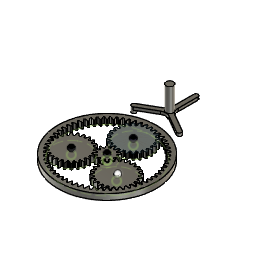
SizeFixedPlanetaryGearShaft (Autodesk Fusion 360 design; units mm, degrees)
description: Spur Gear; Diametrial Pitch: 10.0; Num Teeth: 60; Pressure Angle: 20.0; Backlash: 0.00 in
description: Spur Gear; Diametrial Pitch: 10.0; Num Teeth: 12; Pressure Angle: 20.0; Backlash: 0.00 in
description: Spur Gear; Diametrial Pitch: 10.0; Num Teeth: 24; Pressure Angle: 20.0; Backlash: 0.03 in
Autodesk Fusion 360 part; units mm, degrees
(part 1 of 3)
sketch "Sketch1" plane through (0, 0, 0) normal (0, 0, 1) x (1, 0, 0) in component "Spur Gear (60 teeth)"
  circle A0 centre (0, 0) radius 73.1012
  circle A1 centre (0, 0) radius 1.4986
extrude "Extrude1" add sketch "Sketch1" along normal blind 10.16 makes body 1 in component "Spur Gear (60 teeth)"
sketch "Sketch2" plane through (0, 0, 0) normal (0, 0, 1) x (1, 0, 0) in component "Spur Gear (60 teeth)"
  spline S0 degree 5 poles (71.5442, -2.941) (71.5649, -2.941) (71.6065, -2.9408) (71.6689, -2.94) (71.7521, -2.938) (71.8561, -2.9339) (71.96, -2.9282) (72.064, -2.921) (72.168, -2.9123) (72.272, -2.9022) (72.3759, -2.891) (72.4799, -2.8787) (72.5838, -2.8655) (72.6877, -2.8514) (72.7915, -2.8365) (72.8954, -2.8208) (72.9992, -2.8044) (73.1029, -2.7872) (73.2067, -2.7693) (73.3103, -2.7506) (73.414, -2.7311) (73.5176, -2.711) (73.6212, -2.6902) (73.7248, -2.6688) (73.8283, -2.6468) (73.9317, -2.6241) (74.0351, -2.6008) (74.1385, -2.577) (74.2418, -2.5525) (74.3451, -2.5275) (74.4484, -2.5019) (74.5516, -2.4757) (74.6547, -2.449) (74.7578, -2.4218) (74.8608, -2.394) (74.9638, -2.3657) (75.0668, -2.3369) (75.1697, -2.3075) (75.2725, -2.2777) (75.3753, -2.2474) (75.478, -2.2166) (75.5807, -2.1852) (75.6833, -2.1535) (75.7859, -2.1212) (75.8884, -2.0885) (75.9909, -2.0553) (76.0933, -2.0216) (76.1956, -1.9875) (76.2979, -1.953) (76.4001, -1.918) (76.5023, -1.8825) (76.6044, -1.8466) (76.7064, -1.8103) (76.8084, -1.7736) (76.9103, -1.7364) (77.0122, -1.6988) (77.114, -1.6608) (77.2157, -1.6223) (77.3174, -1.5835) (77.419, -1.5442) (77.5205, -1.5046) (77.622, -1.4645) (77.7234, -1.424) (77.8247, -1.3831) (77.926, -1.3419) (78.0272, -1.3002) (78.1283, -1.2582) (78.2294, -1.2157) (78.3304, -1.1729) (78.4313, -1.1297) (78.5322, -1.0862) (78.6128, -1.051) (78.6733, -1.0244) (78.7135, -1.0067) (78.7337, -0.9978) knots 0 0 0 0 0 0 0.01428571 0.02857143 0.04285714 0.05714286 0.07142857 0.08571429 0.1 0.11428571 0.12857143 0.14285714 0.15714286 0.17142857 0.18571429 0.2 0.21428571 0.22857143 0.24285714 0.25714286 0.27142857 0.28571429 0.3 0.31428571 0.32857143 0.34285714 0.35714286 0.37142857 0.38571429 0.4 0.41428571 0.42857143 0.44285714 0.45714286 0.47142857 0.48571429 0.5 0.51428571 0.52857143 0.54285714 0.55714286 0.57142857 0.58571429 0.6 0.61428571 0.62857143 0.64285714 0.65714286 0.67142857 0.68571429 0.7 0.71428571 0.72857143 0.74285714 0.75714286 0.77142857 0.78571429 0.8 0.81428571 0.82857143 0.84285714 0.85714286 0.87142857 0.88571429 0.9 0.91428571 0.92857143 0.94285714 0.95714286 0.97142857 0.98571429 1 1 1 1 1 1
  spline S1 degree 5 poles (71.5442, 2.941) (71.5649, 2.941) (71.6065, 2.9408) (71.6689, 2.94) (71.7521, 2.938) (71.8561, 2.9339) (71.96, 2.9282) (72.064, 2.921) (72.168, 2.9123) (72.272, 2.9022) (72.3759, 2.891) (72.4799, 2.8787) (72.5838, 2.8655) (72.6877, 2.8514) (72.7915, 2.8365) (72.8954, 2.8208) (72.9992, 2.8044) (73.1029, 2.7872) (73.2067, 2.7693) (73.3103, 2.7506) (73.414, 2.7311) (73.5176, 2.711) (73.6212, 2.6902) (73.7248, 2.6688) (73.8283, 2.6468) (73.9317, 2.6241) (74.0351, 2.6008) (74.1385, 2.577) (74.2418, 2.5525) (74.3451, 2.5275) (74.4484, 2.5019) (74.5516, 2.4757) (74.6547, 2.449) (74.7578, 2.4218) (74.8608, 2.394) (74.9638, 2.3657) (75.0668, 2.3369) (75.1697, 2.3075) (75.2725, 2.2777) (75.3753, 2.2474) (75.478, 2.2166) (75.5807, 2.1852) (75.6833, 2.1535) (75.7859, 2.1212) (75.8884, 2.0885) (75.9909, 2.0553) (76.0933, 2.0216) (76.1956, 1.9875) (76.2979, 1.953) (76.4001, 1.918) (76.5023, 1.8825) (76.6044, 1.8466) (76.7064, 1.8103) (76.8084, 1.7736) (76.9103, 1.7364) (77.0122, 1.6988) (77.114, 1.6608) (77.2157, 1.6223) (77.3174, 1.5835) (77.419, 1.5442) (77.5205, 1.5046) (77.622, 1.4645) (77.7234, 1.424) (77.8247, 1.3831) (77.926, 1.3419) (78.0272, 1.3002) (78.1283, 1.2582) (78.2294, 1.2157) (78.3304, 1.1729) (78.4313, 1.1297) (78.5322, 1.0862) (78.6128, 1.051) (78.6733, 1.0244) (78.7135, 1.0067) (78.7337, 0.9978) knots 0 0 0 0 0 0 0.01428571 0.02857143 0.04285714 0.05714286 0.07142857 0.08571429 0.1 0.11428571 0.12857143 0.14285714 0.15714286 0.17142857 0.18571429 0.2 0.21428571 0.22857143 0.24285714 0.25714286 0.27142857 0.28571429 0.3 0.31428571 0.32857143 0.34285714 0.35714286 0.37142857 0.38571429 0.4 0.41428571 0.42857143 0.44285714 0.45714286 0.47142857 0.48571429 0.5 0.51428571 0.52857143 0.54285714 0.55714286 0.57142857 0.58571429 0.6 0.61428571 0.62857143 0.64285714 0.65714286 0.67142857 0.68571429 0.7 0.71428571 0.72857143 0.74285714 0.75714286 0.77142857 0.78571429 0.8 0.81428571 0.82857143 0.84285714 0.85714286 0.87142857 0.88571429 0.9 0.91428571 0.92857143 0.94285714 0.95714286 0.97142857 0.98571429 1 1 1 1 1 1
  arc A0 (78.7337, -0.9978) -> (78.7337, 0.9978) centre (0, 0) ccw
  line L0 (71.5442, 2.941) -> (71.5442, -2.941)
  point P0 (72.0551, -2.9213)
  point P1 (72.5673, -2.8674)
  point P2 (73.0803, -2.7909)
  point P3 (73.5939, -2.6956)
  point P4 (74.1079, -2.5839)
  point P5 (74.6222, -2.4574)
  point P6 (75.1366, -2.3169)
  point P7 (75.651, -2.1634)
  point P8 (76.1654, -1.9975)
  point P9 (76.6797, -1.8197)
  point P10 (77.1938, -1.6305)
  point P11 (77.7075, -1.4303)
  point P12 (78.2208, -1.2193)
  point P13 (72.0551, 2.9213)
  point P14 (72.5673, 2.8674)
  point P15 (73.0803, 2.7909)
  point P16 (73.5939, 2.6956)
  point P17 (74.1079, 2.5839)
  point P18 (74.6222, 2.4574)
  point P19 (75.1366, 2.3169)
  point P20 (75.651, 2.1634)
  point P21 (76.1654, 1.9975)
  point P22 (76.6797, 1.8197)
  point P23 (77.1938, 1.6305)
  point P24 (77.7075, 1.4303)
  point P25 (78.2208, 1.2193)
extrude "Extrude2" add sketch "Sketch2" along normal blind 10.16 bodies 1 in component "Spur Gear (60 teeth)"
fillet "Fillet1" radius 1.27 2 edges at (73.0477, 2.7963, 5.08) (73.0477, -2.7963, 5.08) on bodies 1 in component "Spur Gear (60 teeth)"
pattern_circular "C-Pattern1" count 60 over 360 about axis through (0, 0, 0) along (0, 0, 1) of "Extrude2", "Fillet1" in component "Spur Gear (60 teeth)"
sketch "Sketch3" plane through (0, 0, 0) normal (0, 0, 1) x (1, 0, 0) in component "Spur Gear (60 teeth)"
  circle A0 centre (0, 0) radius 76.2 construction
sketch "Sketch1 (2)" plane through (0, 0, 0) normal (0, 0, 1) x (1, 0, 0)
  circle A0 centre (0, 0) radius 85.725
  dimension "d12" = 171.45
  constraint coincident A0.centre origin
  measures "d12" diameter of A0
extrude "Extrude1'" add sketch "Sketch1 (2)" along normal blind 10.16 separate body makes body 2
combine "Combine1" operation cut target body 2 tool bodies 1 makes body 3 at (1.4967, -0.0747, 6.7733)
sketch "Sketch2 (2)" plane through (0, 0, 10.16) normal (0, 0, 1) x (-1, 0, 0)
  circle A0 centre (0, 0) radius 1.4986
  circle A1 centre (0, 0) radius 1.4986
  constraint concentric A0 A1
extrude "Extrude2'" cut sketch "Sketch2 (2)" against normal blind 15.24 bodies 3
sketch "Sketch1 (3)" plane through (0, 0, 0) normal (0, 0, 1) x (1, 0, 0) in component "Spur Gear (12 teeth)"
  circle A0 centre (0, 0) radius 12.1412
  circle A1 centre (0, 0) radius 1.4986
extrude "Extrude1''" add sketch "Sketch1 (3)" along normal blind 10.16 separate body makes body 4 in component "Spur Gear (12 teeth)"
sketch "Sketch2 (3)" plane through (0, 0, 0) normal (0, 0, 1) x (1, 0, 0) in component "Spur Gear (12 teeth)"
  spline S0 degree 5 poles (14.169, -2.0807) (14.1792, -2.0821) (14.1996, -2.0848) (14.2302, -2.0878) (14.2713, -2.09) (14.3228, -2.0901) (14.3745, -2.0884) (14.4263, -2.0857) (14.4781, -2.0823) (14.53, -2.0784) (14.582, -2.0742) (14.6339, -2.0693) (14.686, -2.0636) (14.738, -2.057) (14.7901, -2.0496) (14.8422, -2.0413) (14.8944, -2.0323) (14.9466, -2.0226) (14.9987, -2.0125) (15.0509, -2.0018) (15.1031, -1.9907) (15.1552, -1.979) (15.2074, -1.9667) (15.2596, -1.9539) (15.3117, -1.9405) (15.3639, -1.9266) (15.416, -1.9121) (15.4681, -1.8971) (15.5202, -1.8817) (15.5723, -1.8658) (15.6244, -1.8494) (15.6764, -1.8326) (15.7284, -1.8153) (15.7803, -1.7975) (15.8322, -1.7793) (15.8841, -1.7606) (15.936, -1.7415) (15.9878, -1.7219) (16.0396, -1.7019) (16.0913, -1.6814) (16.143, -1.6606) (16.1946, -1.6393) (16.2462, -1.6176) (16.2977, -1.5955) (16.3492, -1.573) (16.4006, -1.5501) (16.452, -1.5268) (16.5033, -1.503) (16.5546, -1.4789) (16.6058, -1.4544) (16.6569, -1.4295) (16.7079, -1.4042) (16.7589, -1.3786) (16.8099, -1.3525) (16.8607, -1.3261) (16.9115, -1.2993) (16.9622, -1.2721) (17.0129, -1.2445) (17.0634, -1.2166) (17.1139, -1.1883) (17.1643, -1.1597) (17.2147, -1.1307) (17.2649, -1.1013) (17.3151, -1.0716) (17.3651, -1.0415) (17.4151, -1.0111) (17.465, -0.9803) (17.5148, -0.9492) (17.5646, -0.9177) (17.6142, -0.8859) (17.6637, -0.8537) (17.7033, -0.8277) (17.7329, -0.8081) (17.7527, -0.7949) (17.7625, -0.7883) knots 0 0 0 0 0 0 0.01428571 0.02857143 0.04285714 0.05714286 0.07142857 0.08571429 0.1 0.11428571 0.12857143 0.14285714 0.15714286 0.17142857 0.18571429 0.2 0.21428571 0.22857143 0.24285714 0.25714286 0.27142857 0.28571429 0.3 0.31428571 0.32857143 0.34285714 0.35714286 0.37142857 0.38571429 0.4 0.41428571 0.42857143 0.44285714 0.45714286 0.47142857 0.48571429 0.5 0.51428571 0.52857143 0.54285714 0.55714286 0.57142857 0.58571429 0.6 0.61428571 0.62857143 0.64285714 0.65714286 0.67142857 0.68571429 0.7 0.71428571 0.72857143 0.74285714 0.75714286 0.77142857 0.78571429 0.8 0.81428571 0.82857143 0.84285714 0.85714286 0.87142857 0.88571429 0.9 0.91428571 0.92857143 0.94285714 0.95714286 0.97142857 0.98571429 1 1 1 1 1 1
  spline S1 degree 5 poles (14.169, 2.0807) (14.1792, 2.0821) (14.1996, 2.0848) (14.2302, 2.0878) (14.2713, 2.09) (14.3228, 2.0901) (14.3745, 2.0884) (14.4263, 2.0857) (14.4781, 2.0823) (14.53, 2.0784) (14.582, 2.0742) (14.6339, 2.0693) (14.686, 2.0636) (14.738, 2.057) (14.7901, 2.0496) (14.8422, 2.0413) (14.8944, 2.0323) (14.9466, 2.0226) (14.9987, 2.0125) (15.0509, 2.0018) (15.1031, 1.9907) (15.1552, 1.979) (15.2074, 1.9667) (15.2596, 1.9539) (15.3117, 1.9405) (15.3639, 1.9266) (15.416, 1.9121) (15.4681, 1.8971) (15.5202, 1.8817) (15.5723, 1.8658) (15.6244, 1.8494) (15.6764, 1.8326) (15.7284, 1.8153) (15.7803, 1.7975) (15.8322, 1.7793) (15.8841, 1.7606) (15.936, 1.7415) (15.9878, 1.7219) (16.0396, 1.7019) (16.0913, 1.6814) (16.143, 1.6606) (16.1946, 1.6393) (16.2462, 1.6176) (16.2977, 1.5955) (16.3492, 1.573) (16.4006, 1.5501) (16.452, 1.5268) (16.5033, 1.503) (16.5546, 1.4789) (16.6058, 1.4544) (16.6569, 1.4295) (16.7079, 1.4042) (16.7589, 1.3786) (16.8099, 1.3525) (16.8607, 1.3261) (16.9115, 1.2993) (16.9622, 1.2721) (17.0129, 1.2445) (17.0634, 1.2166) (17.1139, 1.1883) (17.1643, 1.1597) (17.2147, 1.1307) (17.2649, 1.1013) (17.3151, 1.0716) (17.3651, 1.0415) (17.4151, 1.0111) (17.465, 0.9803) (17.5148, 0.9492) (17.5646, 0.9177) (17.6142, 0.8859) (17.6637, 0.8537) (17.7033, 0.8277) (17.7329, 0.8081) (17.7527, 0.7949) (17.7625, 0.7883) knots 0 0 0 0 0 0 0.01428571 0.02857143 0.04285714 0.05714286 0.07142857 0.08571429 0.1 0.11428571 0.12857143 0.14285714 0.15714286 0.17142857 0.18571429 0.2 0.21428571 0.22857143 0.24285714 0.25714286 0.27142857 0.28571429 0.3 0.31428571 0.32857143 0.34285714 0.35714286 0.37142857 0.38571429 0.4 0.41428571 0.42857143 0.44285714 0.45714286 0.47142857 0.48571429 0.5 0.51428571 0.52857143 0.54285714 0.55714286 0.57142857 0.58571429 0.6 0.61428571 0.62857143 0.64285714 0.65714286 0.67142857 0.68571429 0.7 0.71428571 0.72857143 0.74285714 0.75714286 0.77142857 0.78571429 0.8 0.81428571 0.82857143 0.84285714 0.85714286 0.87142857 0.88571429 0.9 0.91428571 0.92857143 0.94285714 0.95714286 0.97142857 0.98571429 1 1 1 1 1 1
  arc A0 (17.7625, -0.7883) -> (17.7625, 0.7883) centre (0, 0) ccw
  line L0 (12.0025, -1.764) -> (14.169, -2.0807)
  line L1 (12.0025, 1.764) -> (14.169, 2.0807)
  line L2 (12.0025, -1.764) -> (12.0025, 1.764)
  point P0 (14.4179, -2.086)
  point P1 (14.6704, -2.0652)
  point P2 (14.9252, -2.0265)
  point P3 (15.1816, -1.9727)
  point P4 (15.4392, -1.9054)
  point P5 (15.6976, -1.8255)
  point P6 (15.9566, -1.7336)
  point P7 (16.2158, -1.6304)
  point P8 (16.475, -1.5161)
  point P9 (16.734, -1.3911)
  point P10 (16.9924, -1.2556)
  point P11 (17.2502, -1.1099)
  point P12 (17.5069, -0.954)
  point P13 (14.4179, 2.086)
  point P14 (14.6704, 2.0652)
  point P15 (14.9252, 2.0265)
  point P16 (15.1816, 1.9727)
  point P17 (15.4392, 1.9054)
  point P18 (15.6976, 1.8255)
  point P19 (15.9566, 1.7336)
  point P20 (16.2158, 1.6304)
  point P21 (16.475, 1.5161)
  point P22 (16.734, 1.3911)
  point P23 (16.9924, 1.2556)
  point P24 (17.2502, 1.1099)
  point P25 (17.5069, 0.954)
extrude "Extrude2''" add sketch "Sketch2 (3)" along normal blind 10.16 bodies 4 in component "Spur Gear (12 teeth)"
fillet "Fillet1'" radius 1.27 2 edges at (12.0122, -1.7654, 5.08) (12.0122, 1.7654, 5.08) on bodies 4 in component "Spur Gear (12 teeth)"
pattern_circular "C-Pattern1'" count 12 over 360 about axis through (0, 0, 0) along (0, 0, 1) of "Extrude2''", "Fillet1'" in component "Spur Gear (12 teeth)"
sketch "Sketch3 (2)" plane through (0, 0, 0) normal (0, 0, 1) x (1, 0, 0) in component "Spur Gear (12 teeth)"
  circle A0 centre (0, 0) radius 15.24 construction
sketch "Sketch1 (4)" plane through (0, 0, 0) normal (0, 0, 1) x (1, 0, 0) in component "Spur Gear (24 teeth)"
  circle A0 centre (0, 0) radius 27.3812
  circle A1 centre (0, 0) radius 1.4986
extrude "Extrude1'''" add sketch "Sketch1 (4)" along normal blind 10.16 separate body makes body 5 in component "Spur Gear (24 teeth)"
sketch "Sketch2 (4)" plane through (0, 0, 0) normal (0, 0, 1) x (1, 0, 0) in component "Spur Gear (24 teeth)"
  spline S0 degree 5 poles (28.5632, -2.1205) (28.5761, -2.1215) (28.6017, -2.1231) (28.6403, -2.1244) (28.6917, -2.1245) (28.756, -2.122) (28.8203, -2.1177) (28.8847, -2.1123) (28.9491, -2.1063) (29.0135, -2.0998) (29.078, -2.093) (29.1424, -2.0855) (29.2069, -2.0773) (29.2713, -2.0683) (29.3357, -2.0583) (29.4002, -2.0476) (29.4646, -2.0361) (29.529, -2.0241) (29.5934, -2.0115) (29.6577, -1.9985) (29.7221, -1.985) (29.7864, -1.971) (29.8507, -1.9565) (29.915, -1.9414) (29.9792, -1.9257) (30.0435, -1.9096) (30.1077, -1.893) (30.1718, -1.8759) (30.236, -1.8583) (30.3001, -1.8403) (30.3642, -1.8219) (30.4282, -1.803) (30.4922, -1.7837) (30.5562, -1.7639) (30.6201, -1.7437) (30.684, -1.7231) (30.7478, -1.7021) (30.8117, -1.6807) (30.8754, -1.6589) (30.9392, -1.6367) (31.0028, -1.614) (31.0665, -1.591) (31.1301, -1.5677) (31.1936, -1.5439) (31.2571, -1.5197) (31.3206, -1.4952) (31.384, -1.4703) (31.4473, -1.4451) (31.5106, -1.4194) (31.5739, -1.3935) (31.6371, -1.3671) (31.7002, -1.3404) (31.7633, -1.3134) (31.8264, -1.286) (31.8893, -1.2582) (31.9523, -1.2301) (32.0151, -1.2017) (32.0779, -1.1729) (32.1407, -1.1438) (32.2034, -1.1144) (32.266, -1.0846) (32.3286, -1.0546) (32.3911, -1.0241) (32.4535, -0.9934) (32.5159, -0.9623) (32.5782, -0.9309) (32.6405, -0.8992) (32.7026, -0.8672) (32.7648, -0.8349) (32.8268, -0.8022) (32.8888, -0.7693) (32.9383, -0.7426) (32.9754, -0.7225) (33.0002, -0.7091) (33.0125, -0.7023) knots 0 0 0 0 0 0 0.01428571 0.02857143 0.04285714 0.05714286 0.07142857 0.08571429 0.1 0.11428571 0.12857143 0.14285714 0.15714286 0.17142857 0.18571429 0.2 0.21428571 0.22857143 0.24285714 0.25714286 0.27142857 0.28571429 0.3 0.31428571 0.32857143 0.34285714 0.35714286 0.37142857 0.38571429 0.4 0.41428571 0.42857143 0.44285714 0.45714286 0.47142857 0.48571429 0.5 0.51428571 0.52857143 0.54285714 0.55714286 0.57142857 0.58571429 0.6 0.61428571 0.62857143 0.64285714 0.65714286 0.67142857 0.68571429 0.7 0.71428571 0.72857143 0.74285714 0.75714286 0.77142857 0.78571429 0.8 0.81428571 0.82857143 0.84285714 0.85714286 0.87142857 0.88571429 0.9 0.91428571 0.92857143 0.94285714 0.95714286 0.97142857 0.98571429 1 1 1 1 1 1
  spline S1 degree 5 poles (28.5632, 2.1205) (28.5761, 2.1215) (28.6017, 2.1231) (28.6403, 2.1244) (28.6917, 2.1245) (28.756, 2.122) (28.8203, 2.1177) (28.8847, 2.1123) (28.9491, 2.1063) (29.0135, 2.0998) (29.078, 2.093) (29.1424, 2.0855) (29.2069, 2.0773) (29.2713, 2.0683) (29.3357, 2.0583) (29.4002, 2.0476) (29.4646, 2.0361) (29.529, 2.0241) (29.5934, 2.0115) (29.6577, 1.9985) (29.7221, 1.985) (29.7864, 1.971) (29.8507, 1.9565) (29.915, 1.9414) (29.9792, 1.9257) (30.0435, 1.9096) (30.1077, 1.893) (30.1718, 1.8759) (30.236, 1.8583) (30.3001, 1.8403) (30.3642, 1.8219) (30.4282, 1.803) (30.4922, 1.7837) (30.5562, 1.7639) (30.6201, 1.7437) (30.684, 1.7231) (30.7478, 1.7021) (30.8117, 1.6807) (30.8754, 1.6589) (30.9392, 1.6367) (31.0028, 1.614) (31.0665, 1.591) (31.1301, 1.5677) (31.1936, 1.5439) (31.2571, 1.5197) (31.3206, 1.4952) (31.384, 1.4703) (31.4473, 1.4451) (31.5106, 1.4194) (31.5739, 1.3935) (31.6371, 1.3671) (31.7002, 1.3404) (31.7633, 1.3134) (31.8264, 1.286) (31.8893, 1.2582) (31.9523, 1.2301) (32.0151, 1.2017) (32.0779, 1.1729) (32.1407, 1.1438) (32.2034, 1.1144) (32.266, 1.0846) (32.3286, 1.0546) (32.3911, 1.0241) (32.4535, 0.9934) (32.5159, 0.9623) (32.5782, 0.9309) (32.6405, 0.8992) (32.7026, 0.8672) (32.7648, 0.8349) (32.8268, 0.8022) (32.8888, 0.7693) (32.9383, 0.7426) (32.9754, 0.7225) (33.0002, 0.7091) (33.0125, 0.7023) knots 0 0 0 0 0 0 0.01428571 0.02857143 0.04285714 0.05714286 0.07142857 0.08571429 0.1 0.11428571 0.12857143 0.14285714 0.15714286 0.17142857 0.18571429 0.2 0.21428571 0.22857143 0.24285714 0.25714286 0.27142857 0.28571429 0.3 0.31428571 0.32857143 0.34285714 0.35714286 0.37142857 0.38571429 0.4 0.41428571 0.42857143 0.44285714 0.45714286 0.47142857 0.48571429 0.5 0.51428571 0.52857143 0.54285714 0.55714286 0.57142857 0.58571429 0.6 0.61428571 0.62857143 0.64285714 0.65714286 0.67142857 0.68571429 0.7 0.71428571 0.72857143 0.74285714 0.75714286 0.77142857 0.78571429 0.8 0.81428571 0.82857143 0.84285714 0.85714286 0.87142857 0.88571429 0.9 0.91428571 0.92857143 0.94285714 0.95714286 0.97142857 0.98571429 1 1 1 1 1 1
  arc A0 (33.0125, -0.7023) -> (33.0125, 0.7023) centre (0, 0) ccw
  line L0 (27.2961, -2.0272) -> (28.5632, -2.1205)
  line L1 (27.2961, 2.0272) -> (28.5632, 2.1205)
  line L2 (27.2961, -2.0272) -> (27.2961, 2.0272)
  point P0 (28.8774, -2.1128)
  point P1 (29.1934, -2.0789)
  point P2 (29.5104, -2.0275)
  point P3 (29.8283, -1.9614)
  point P4 (30.1467, -1.8825)
  point P5 (30.4656, -1.7917)
  point P6 (30.7846, -1.6897)
  point P7 (31.1037, -1.5773)
  point P8 (31.4227, -1.4548)
  point P9 (31.7415, -1.3227)
  point P10 (32.0601, -1.1811)
  point P11 (32.3782, -1.0304)
  point P12 (32.6957, -0.8707)
  point P13 (28.8774, 2.1128)
  point P14 (29.1934, 2.0789)
  point P15 (29.5104, 2.0275)
  point P16 (29.8283, 1.9614)
  point P17 (30.1467, 1.8825)
  point P18 (30.4656, 1.7917)
  point P19 (30.7846, 1.6897)
  point P20 (31.1037, 1.5773)
  point P21 (31.4227, 1.4548)
  point P22 (31.7415, 1.3227)
  point P23 (32.0601, 1.1811)
  point P24 (32.3782, 1.0304)
  point P25 (32.6957, 0.8707)
extrude "Extrude2'''" add sketch "Sketch2 (4)" along normal blind 10.16 bodies 5 in component "Spur Gear (24 teeth)"
fillet "Fillet1''" radius 1.27 2 edges at (27.306, -2.0279, 5.08) (27.306, 2.0279, 5.08) on bodies 5 in component "Spur Gear (24 teeth)"
pattern_circular "C-Pattern1''" count 24 over 360 about axis through (0, 0, 0) along (0, 0, 1) of "Extrude2'''", "Fillet1''" in component "Spur Gear (24 teeth)"
sketch "Sketch3 (3)" plane through (0, 0, 0) normal (0, 0, 1) x (1, 0, 0) in component "Spur Gear (24 teeth)"
  circle A0 centre (0, 0) radius 30.48 construction
sketch "Sketch3 (4)" plane through (0, 0, 10.16) normal (0, 0, 1) x (-1, 0, 0)
  arc A0 (-27.1003, -41.8082) -> (-27.1894, -42.4844) centre (0, -45.72) ccw
  arc A1 (-28.5437, -43.6009) -> (-27.1894, -42.4844) centre (-28.4505, -42.3343) ccw
  line L0 (-28.5437, -43.6009) -> (-28.5632, -43.5995)
  spline S0 degree 5 poles (-28.5632, -43.5995) (-28.5761, -43.5985) (-28.6017, -43.5969) (-28.6403, -43.5956) (-28.6917, -43.5955) (-28.756, -43.598) (-28.8203, -43.6023) (-28.8847, -43.6077) (-28.9491, -43.6137) (-29.0135, -43.6202) (-29.078, -43.627) (-29.1424, -43.6345) (-29.2069, -43.6427) (-29.2713, -43.6517) (-29.3357, -43.6617) (-29.4002, -43.6724) (-29.4646, -43.6839) (-29.529, -43.6959) (-29.5934, -43.7085) (-29.6577, -43.7215) (-29.7221, -43.735) (-29.7864, -43.749) (-29.8507, -43.7635) (-29.915, -43.7786) (-29.9792, -43.7943) (-30.0435, -43.8104) (-30.1077, -43.827) (-30.1718, -43.8441) (-30.236, -43.8617) (-30.3001, -43.8797) (-30.3642, -43.8981) (-30.4282, -43.917) (-30.4922, -43.9363) (-30.5562, -43.9561) (-30.6201, -43.9763) (-30.684, -43.9969) (-30.7478, -44.0179) (-30.8117, -44.0393) (-30.8754, -44.0611) (-30.9392, -44.0833) (-31.0028, -44.106) (-31.0665, -44.129) (-31.1301, -44.1523) (-31.1936, -44.1761) (-31.2571, -44.2003) (-31.3206, -44.2248) (-31.384, -44.2497) (-31.4473, -44.2749) (-31.5106, -44.3006) (-31.5739, -44.3265) (-31.6371, -44.3529) (-31.7002, -44.3796) (-31.7633, -44.4066) (-31.8264, -44.434) (-31.8893, -44.4618) (-31.9523, -44.4899) (-32.0151, -44.5183) (-32.0779, -44.5471) (-32.1407, -44.5762) (-32.2034, -44.6056) (-32.266, -44.6354) (-32.3286, -44.6654) (-32.3911, -44.6959) (-32.4535, -44.7266) (-32.5159, -44.7577) (-32.5782, -44.7891) (-32.6405, -44.8208) (-32.7026, -44.8528) (-32.7648, -44.8851) (-32.8268, -44.9178) (-32.8888, -44.9507) (-32.9383, -44.9774) (-32.9754, -44.9975) (-33.0002, -45.0109) (-33.0125, -45.0177) knots 0 0 0 0 0 0 0.01428571 0.02857143 0.04285714 0.05714286 0.07142857 0.08571429 0.1 0.11428571 0.12857143 0.14285714 0.15714286 0.17142857 0.18571429 0.2 0.21428571 0.22857143 0.24285714 0.25714286 0.27142857 0.28571429 0.3 0.31428571 0.32857143 0.34285714 0.35714286 0.37142857 0.38571429 0.4 0.41428571 0.42857143 0.44285714 0.45714286 0.47142857 0.48571429 0.5 0.51428571 0.52857143 0.54285714 0.55714286 0.57142857 0.58571429 0.6 0.61428571 0.62857143 0.64285714 0.65714286 0.67142857 0.68571429 0.7 0.71428571 0.72857143 0.74285714 0.75714286 0.77142857 0.78571429 0.8 0.81428571 0.82857143 0.84285714 0.85714286 0.87142857 0.88571429 0.9 0.91428571 0.92857143 0.94285714 0.95714286 0.97142857 0.98571429 1 1 1 1 1 1
  arc A2 (-33.0125, -45.0177) -> (-33.0125, -46.4223) centre (0, -45.72) ccw
  spline S1 degree 5 poles (-33.0125, -46.4223) (-33.0002, -46.4291) (-32.9754, -46.4425) (-32.9383, -46.4626) (-32.8888, -46.4893) (-32.8268, -46.5222) (-32.7648, -46.5549) (-32.7026, -46.5872) (-32.6405, -46.6192) (-32.5782, -46.6509) (-32.5159, -46.6823) (-32.4535, -46.7134) (-32.3911, -46.7441) (-32.3286, -46.7746) (-32.266, -46.8046) (-32.2034, -46.8344) (-32.1407, -46.8638) (-32.0779, -46.8929) (-32.0151, -46.9217) (-31.9523, -46.9501) (-31.8893, -46.9782) (-31.8264, -47.006) (-31.7633, -47.0334) (-31.7002, -47.0604) (-31.6371, -47.0871) (-31.5739, -47.1135) (-31.5106, -47.1394) (-31.4473, -47.1651) (-31.384, -47.1903) (-31.3206, -47.2152) (-31.2571, -47.2397) (-31.1936, -47.2639) (-31.1301, -47.2877) (-31.0665, -47.311) (-31.0028, -47.334) (-30.9392, -47.3567) (-30.8754, -47.3789) (-30.8117, -47.4007) (-30.7478, -47.4221) (-30.684, -47.4431) (-30.6201, -47.4637) (-30.5562, -47.4839) (-30.4922, -47.5037) (-30.4282, -47.523) (-30.3642, -47.5419) (-30.3001, -47.5603) (-30.236, -47.5783) (-30.1718, -47.5959) (-30.1077, -47.613) (-30.0435, -47.6296) (-29.9792, -47.6457) (-29.915, -47.6614) (-29.8507, -47.6765) (-29.7864, -47.691) (-29.7221, -47.705) (-29.6577, -47.7185) (-29.5934, -47.7315) (-29.529, -47.7441) (-29.4646, -47.7561) (-29.4002, -47.7676) (-29.3357, -47.7783) (-29.2713, -47.7883) (-29.2069, -47.7973) (-29.1424, -47.8055) (-29.078, -47.813) (-29.0135, -47.8198) (-28.9491, -47.8263) (-28.8847, -47.8323) (-28.8203, -47.8377) (-28.756, -47.842) (-28.6917, -47.8445) (-28.6403, -47.8444) (-28.6017, -47.8431) (-28.5761, -47.8415) (-28.5632, -47.8405) knots -1 -1 -1 -1 -1 -1 -0.98571429 -0.97142857 -0.95714286 -0.94285714 -0.92857143 -0.91428571 -0.9 -0.88571429 -0.87142857 -0.85714286 -0.84285714 -0.82857143 -0.81428571 -0.8 -0.78571429 -0.77142857 -0.75714286 -0.74285714 -0.72857143 -0.71428571 -0.7 -0.68571429 -0.67142857 -0.65714286 -0.64285714 -0.62857143 -0.61428571 -0.6 -0.58571429 -0.57142857 -0.55714286 -0.54285714 -0.52857143 -0.51428571 -0.5 -0.48571429 -0.47142857 -0.45714286 -0.44285714 -0.42857143 -0.41428571 -0.4 -0.38571429 -0.37142857 -0.35714286 -0.34285714 -0.32857143 -0.31428571 -0.3 -0.28571429 -0.27142857 -0.25714286 -0.24285714 -0.22857143 -0.21428571 -0.2 -0.18571429 -0.17142857 -0.15714286 -0.14285714 -0.12857143 -0.11428571 -0.1 -0.08571429 -0.07142857 -0.05714286 -0.04285714 -0.02857143 -0.01428571 0 0 0 0 0 0
  line L1 (-28.5632, -47.8405) -> (-28.5437, -47.8391)
  arc A3 (-27.1894, -48.9556) -> (-28.5437, -47.8391) centre (-28.4505, -49.1057) ccw
  arc A4 (-27.1894, -48.9556) -> (-27.1003, -49.6318) centre (0, -45.72) ccw
  arc A5 (-28.1196, -51.0608) -> (-27.1003, -49.6318) centre (-28.3573, -49.8132) ccw
  line L2 (-28.1196, -51.0608) -> (-28.1388, -51.0644)
  spline S2 degree 5 poles (-28.1388, -51.0644) (-28.1514, -51.0668) (-28.1766, -51.072) (-28.2142, -51.0806) (-28.2639, -51.0939) (-28.3253, -51.1129) (-28.3864, -51.1337) (-28.4472, -51.1556) (-28.5078, -51.1781) (-28.5684, -51.201) (-28.6289, -51.2243) (-28.6892, -51.2482) (-28.7493, -51.2728) (-28.8092, -51.2982) (-28.8689, -51.3245) (-28.9283, -51.3515) (-28.9876, -51.3792) (-29.0467, -51.4075) (-29.1056, -51.4363) (-29.1644, -51.4656) (-29.2231, -51.4953) (-29.2816, -51.5254) (-29.3399, -51.5561) (-29.3981, -51.5873) (-29.4561, -51.6191) (-29.514, -51.6513) (-29.5717, -51.684) (-29.6293, -51.7171) (-29.6867, -51.7507) (-29.7439, -51.7846) (-29.8011, -51.819) (-29.858, -51.8538) (-29.9149, -51.8891) (-29.9715, -51.9247) (-30.0281, -51.9607) (-30.0844, -51.9972) (-30.1407, -52.034) (-30.1968, -52.0712) (-30.2527, -52.1088) (-30.3085, -52.1468) (-30.3642, -52.1851) (-30.4197, -52.2238) (-30.4751, -52.2628) (-30.5303, -52.3022) (-30.5854, -52.342) (-30.6404, -52.3821) (-30.6952, -52.4226) (-30.7498, -52.4633) (-30.8043, -52.5045) (-30.8587, -52.546) (-30.9129, -52.5878) (-30.967, -52.6299) (-31.0209, -52.6723) (-31.0747, -52.7151) (-31.1284, -52.7582) (-31.1819, -52.8016) (-31.2353, -52.8454) (-31.2885, -52.8894) (-31.3416, -52.9338) (-31.3945, -52.9784) (-31.4473, -53.0234) (-31.4999, -53.0686) (-31.5524, -53.1142) (-31.6048, -53.1601) (-31.657, -53.2062) (-31.7091, -53.2527) (-31.761, -53.2994) (-31.8128, -53.3464) (-31.8644, -53.3937) (-31.9159, -53.4413) (-31.9672, -53.4892) (-32.0082, -53.5277) (-32.0388, -53.5568) (-32.0592, -53.5762) (-32.0694, -53.5859) knots 0 0 0 0 0 0 0.01428571 0.02857143 0.04285714 0.05714286 0.07142857 0.08571429 0.1 0.11428571 0.12857143 0.14285714 0.15714286 0.17142857 0.18571429 0.2 0.21428571 0.22857143 0.24285714 0.25714286 0.27142857 0.28571429 0.3 0.31428571 0.32857143 0.34285714 0.35714286 0.37142857 0.38571429 0.4 0.41428571 0.42857143 0.44285714 0.45714286 0.47142857 0.48571429 0.5 0.51428571 0.52857143 0.54285714 0.55714286 0.57142857 0.58571429 0.6 0.61428571 0.62857143 0.64285714 0.65714286 0.67142857 0.68571429 0.7 0.71428571 0.72857143 0.74285714 0.75714286 0.77142857 0.78571429 0.8 0.81428571 0.82857143 0.84285714 0.85714286 0.87142857 0.88571429 0.9 0.91428571 0.92857143 0.94285714 0.95714286 0.97142857 0.98571429 1 1 1 1 1 1
  arc A6 (-32.0694, -53.5859) -> (-31.7059, -54.9427) centre (0, -45.72) ccw
  spline S3 degree 5 poles (-31.7059, -54.9427) (-31.6922, -54.946) (-31.6648, -54.9526) (-31.6238, -54.9624) (-31.569, -54.9753) (-31.5006, -54.9911) (-31.4322, -55.0066) (-31.3639, -55.0217) (-31.2955, -55.0366) (-31.2272, -55.0511) (-31.1589, -55.0653) (-31.0906, -55.0791) (-31.0223, -55.0927) (-30.9541, -55.1059) (-30.8858, -55.1187) (-30.8176, -55.1313) (-30.7495, -55.1435) (-30.6813, -55.1554) (-30.6132, -55.1669) (-30.5451, -55.1781) (-30.4771, -55.1889) (-30.4091, -55.1994) (-30.3411, -55.2096) (-30.2732, -55.2194) (-30.2053, -55.2288) (-30.1374, -55.2379) (-30.0696, -55.2466) (-30.0018, -55.255) (-29.9341, -55.263) (-29.8664, -55.2706) (-29.7987, -55.2779) (-29.7311, -55.2848) (-29.6636, -55.2913) (-29.5961, -55.2974) (-29.5287, -55.3032) (-29.4613, -55.3085) (-29.394, -55.3135) (-29.3268, -55.3181) (-29.2596, -55.3223) (-29.1925, -55.326) (-29.1254, -55.3294) (-29.0585, -55.3323) (-28.9916, -55.3349) (-28.9247, -55.3369) (-28.858, -55.3386) (-28.7913, -55.3398) (-28.7247, -55.3406) (-28.6582, -55.341) (-28.5918, -55.3409) (-28.5255, -55.3404) (-28.4593, -55.3393) (-28.3932, -55.3378) (-28.3272, -55.3357) (-28.2613, -55.3331) (-28.1956, -55.33) (-28.1299, -55.3264) (-28.0644, -55.3223) (-27.9989, -55.3178) (-27.9336, -55.3127) (-27.8684, -55.3071) (-27.8034, -55.3008) (-27.7386, -55.2938) (-27.674, -55.2858) (-27.6097, -55.2771) (-27.5455, -55.2676) (-27.4815, -55.2575) (-27.4176, -55.2471) (-27.3538, -55.2362) (-27.2902, -55.2248) (-27.2269, -55.2123) (-27.1642, -55.198) (-27.1145, -55.1847) (-27.0777, -55.1734) (-27.0533, -55.1652) (-27.0411, -55.161) knots -1 -1 -1 -1 -1 -1 -0.98571429 -0.97142857 -0.95714286 -0.94285714 -0.92857143 -0.91428571 -0.9 -0.88571429 -0.87142857 -0.85714286 -0.84285714 -0.82857143 -0.81428571 -0.8 -0.78571429 -0.77142857 -0.75714286 -0.74285714 -0.72857143 -0.71428571 -0.7 -0.68571429 -0.67142857 -0.65714286 -0.64285714 -0.62857143 -0.61428571 -0.6 -0.58571429 -0.57142857 -0.55714286 -0.54285714 -0.52857143 -0.51428571 -0.5 -0.48571429 -0.47142857 -0.45714286 -0.44285714 -0.42857143 -0.41428571 -0.4 -0.38571429 -0.37142857 -0.35714286 -0.34285714 -0.32857143 -0.31428571 -0.3 -0.28571429 -0.27142857 -0.25714286 -0.24285714 -0.22857143 -0.21428571 -0.2 -0.18571429 -0.17142857 -0.15714286 -0.14285714 -0.12857143 -0.11428571 -0.1 -0.08571429 -0.07142857 -0.05714286 -0.04285714 -0.02857143 -0.01428571 0 0 0 0 0 0
  line L3 (-27.0411, -55.161) -> (-27.0227, -55.1546)
  arc A7 (-25.4255, -55.8825) -> (-27.0227, -55.1546) centre (-26.6048, -56.3538) ccw
  arc A8 (-25.4255, -55.8825) -> (-25.1645, -56.5126) centre (0, -45.72) ccw
  arc A9 (-25.7792, -58.1567) -> (-25.1645, -56.5126) centre (-26.3317, -57.0131) ccw
  line L4 (-25.7792, -58.1567) -> (-25.7967, -58.1652)
  spline S4 degree 5 poles (-25.7967, -58.1652) (-25.8083, -58.1708) (-25.8314, -58.1822) (-25.8654, -58.2003) (-25.9099, -58.226) (-25.9644, -58.2603) (-26.018, -58.2962) (-26.071, -58.3331) (-26.1238, -58.3705) (-26.1764, -58.4083) (-26.2288, -58.4464) (-26.2808, -58.4851) (-26.3326, -58.5244) (-26.3838, -58.5645) (-26.4347, -58.6053) (-26.4851, -58.6468) (-26.5351, -58.689) (-26.5849, -58.7316) (-26.6344, -58.7746) (-26.6836, -58.8181) (-26.7326, -58.862) (-26.7813, -58.9063) (-26.8297, -58.951) (-26.8778, -58.9962) (-26.9257, -59.0419) (-26.9732, -59.088) (-27.0205, -59.1345) (-27.0675, -59.1814) (-27.1143, -59.2287) (-27.1608, -59.2763) (-27.2071, -59.3243) (-27.2531, -59.3727) (-27.2989, -59.4214) (-27.3444, -59.4705) (-27.3897, -59.5199) (-27.4347, -59.5697) (-27.4795, -59.6198) (-27.524, -59.6703) (-27.5683, -59.7211) (-27.6124, -59.7722) (-27.6563, -59.8236) (-27.6999, -59.8754) (-27.7433, -59.9274) (-27.7864, -59.9798) (-27.8293, -60.0324) (-27.872, -60.0854) (-27.9145, -60.1387) (-27.9567, -60.1922) (-27.9987, -60.2461) (-28.0405, -60.3002) (-28.0821, -60.3546) (-28.1234, -60.4093) (-28.1645, -60.4643) (-28.2054, -60.5195) (-28.2461, -60.575) (-28.2865, -60.6308) (-28.3268, -60.6869) (-28.3668, -60.7432) (-28.4066, -60.7997) (-28.4461, -60.8566) (-28.4855, -60.9137) (-28.5246, -60.971) (-28.5636, -61.0286) (-28.6023, -61.0865) (-28.6408, -61.1446) (-28.679, -61.2029) (-28.7171, -61.2615) (-28.7549, -61.3203) (-28.7925, -61.3794) (-28.83, -61.4387) (-28.8672, -61.4982) (-28.8967, -61.546) (-28.9188, -61.582) (-28.9335, -61.606) (-28.9409, -61.618) knots 0 0 0 0 0 0 0.01428571 0.02857143 0.04285714 0.05714286 0.07142857 0.08571429 0.1 0.11428571 0.12857143 0.14285714 0.15714286 0.17142857 0.18571429 0.2 0.21428571 0.22857143 0.24285714 0.25714286 0.27142857 0.28571429 0.3 0.31428571 0.32857143 0.34285714 0.35714286 0.37142857 0.38571429 0.4 0.41428571 0.42857143 0.44285714 0.45714286 0.47142857 0.48571429 0.5 0.51428571 0.52857143 0.54285714 0.55714286 0.57142857 0.58571429 0.6 0.61428571 0.62857143 0.64285714 0.65714286 0.67142857 0.68571429 0.7 0.71428571 0.72857143 0.74285714 0.75714286 0.77142857 0.78571429 0.8 0.81428571 0.82857143 0.84285714 0.85714286 0.87142857 0.88571429 0.9 0.91428571 0.92857143 0.94285714 0.95714286 0.97142857 0.98571429 1 1 1 1 1 1
  arc A10 (-28.9409, -61.618) -> (-28.2385, -62.8345) centre (0, -45.72) ccw
  spline S5 degree 5 poles (-28.2385, -62.8345) (-28.2244, -62.8342) (-28.1963, -62.8334) (-28.1541, -62.8323) (-28.0979, -62.8306) (-28.0277, -62.8281) (-27.9577, -62.8254) (-27.8877, -62.8223) (-27.8179, -62.819) (-27.7481, -62.8153) (-27.6784, -62.8113) (-27.6089, -62.8071) (-27.5394, -62.8025) (-27.4701, -62.7976) (-27.4009, -62.7923) (-27.3317, -62.7868) (-27.2627, -62.7809) (-27.1938, -62.7748) (-27.1251, -62.7683) (-27.0564, -62.7615) (-26.9879, -62.7543) (-26.9195, -62.7469) (-26.8512, -62.7391) (-26.783, -62.731) (-26.715, -62.7225) (-26.6471, -62.7137) (-26.5793, -62.7046) (-26.5117, -62.6951) (-26.4442, -62.6853) (-26.3768, -62.6752) (-26.3096, -62.6647) (-26.2425, -62.6539) (-26.1756, -62.6427) (-26.1088, -62.6311) (-26.0422, -62.6192) (-25.9758, -62.607) (-25.9095, -62.5943) (-25.8433, -62.5814) (-25.7774, -62.568) (-25.7115, -62.5543) (-25.6459, -62.5402) (-25.5805, -62.5257) (-25.5152, -62.5108) (-25.4501, -62.4955) (-25.3852, -62.4799) (-25.3205, -62.4638) (-25.256, -62.4473) (-25.1916, -62.4305) (-25.1275, -62.4132) (-25.0636, -62.3955) (-24.9999, -62.3774) (-24.9364, -62.3588) (-24.8732, -62.3397) (-24.8103, -62.3201) (-24.7476, -62.3001) (-24.6851, -62.2796) (-24.6228, -62.2587) (-24.5608, -62.2374) (-24.499, -62.2156) (-24.4375, -62.1933) (-24.3763, -62.1704) (-24.3156, -62.1468) (-24.2552, -62.1224) (-24.1953, -62.0973) (-24.1358, -62.0715) (-24.0766, -62.0453) (-24.0175, -62.0186) (-23.9587, -61.9917) (-23.9003, -61.9641) (-23.8424, -61.9357) (-23.7855, -61.9057) (-23.741, -61.88) (-23.7083, -61.8595) (-23.6868, -61.8453) (-23.6762, -61.8381) knots -1 -1 -1 -1 -1 -1 -0.98571429 -0.97142857 -0.95714286 -0.94285714 -0.92857143 -0.91428571 -0.9 -0.88571429 -0.87142857 -0.85714286 -0.84285714 -0.82857143 -0.81428571 -0.8 -0.78571429 -0.77142857 -0.75714286 -0.74285714 -0.72857143 -0.71428571 -0.7 -0.68571429 -0.67142857 -0.65714286 -0.64285714 -0.62857143 -0.61428571 -0.6 -0.58571429 -0.57142857 -0.55714286 -0.54285714 -0.52857143 -0.51428571 -0.5 -0.48571429 -0.47142857 -0.45714286 -0.44285714 -0.42857143 -0.41428571 -0.4 -0.38571429 -0.37142857 -0.35714286 -0.34285714 -0.32857143 -0.31428571 -0.3 -0.28571429 -0.27142857 -0.25714286 -0.24285714 -0.22857143 -0.21428571 -0.2 -0.18571429 -0.17142857 -0.15714286 -0.14285714 -0.12857143 -0.11428571 -0.1 -0.08571429 -0.07142857 -0.05714286 -0.04285714 -0.02857143 -0.01428571 0 0 0 0 0 0
  line L5 (-23.6762, -61.8381) -> (-23.6601, -61.8271)
  arc A11 (-21.9289, -62.1168) -> (-23.6601, -61.8271) centre (-22.946, -62.8773) ccw
  arc A12 (-21.9289, -62.1168) -> (-21.5137, -62.6579) centre (0, -45.72) ccw
  arc A13 (-21.6819, -64.405) -> (-21.5137, -62.6579) centre (-22.5115, -63.4435) ccw
  line L6 (-21.6819, -64.405) -> (-21.6967, -64.4178)
  spline S6 degree 5 poles (-21.6967, -64.4178) (-21.7064, -64.4262) (-21.7257, -64.4433) (-21.7539, -64.4695) (-21.7903, -64.5058) (-21.834, -64.5531) (-21.8765, -64.6016) (-21.9182, -64.651) (-21.9595, -64.7008) (-22.0005, -64.7509) (-22.0412, -64.8013) (-22.0815, -64.8521) (-22.1213, -64.9035) (-22.1604, -64.9555) (-22.199, -65.008) (-22.2369, -65.0612) (-22.2744, -65.1148) (-22.3114, -65.1689) (-22.348, -65.2233) (-22.3843, -65.278) (-22.4203, -65.3331) (-22.4559, -65.3885) (-22.4911, -65.4442) (-22.5258, -65.5003) (-22.5602, -65.5568) (-22.5942, -65.6136) (-22.6279, -65.6708) (-22.6611, -65.7283) (-22.6941, -65.786) (-22.7267, -65.8441) (-22.7589, -65.9025) (-22.7909, -65.9611) (-22.8225, -66.02) (-22.8538, -66.0792) (-22.8847, -66.1387) (-22.9153, -66.1984) (-22.9456, -66.2584) (-22.9756, -66.3187) (-23.0052, -66.3792) (-23.0346, -66.44) (-23.0636, -66.501) (-23.0924, -66.5623) (-23.1208, -66.6238) (-23.1489, -66.6855) (-23.1767, -66.7475) (-23.2043, -66.8097) (-23.2315, -66.8722) (-23.2584, -66.9348) (-23.2851, -66.9977) (-23.3114, -67.0608) (-23.3375, -67.1241) (-23.3633, -67.1876) (-23.3888, -67.2514) (-23.414, -67.3153) (-23.4389, -67.3795) (-23.4635, -67.4438) (-23.4879, -67.5084) (-23.5119, -67.5731) (-23.5357, -67.6381) (-23.5592, -67.7032) (-23.5825, -67.7686) (-23.6054, -67.8341) (-23.6281, -67.8998) (-23.6505, -67.9657) (-23.6727, -68.0318) (-23.6945, -68.098) (-23.7161, -68.1644) (-23.7375, -68.2311) (-23.7585, -68.2978) (-23.7793, -68.3648) (-23.7998, -68.4319) (-23.816, -68.4858) (-23.8281, -68.5262) (-23.836, -68.5533) (-23.84, -68.5668) knots 0 0 0 0 0 0 0.01428571 0.02857143 0.04285714 0.05714286 0.07142857 0.08571429 0.1 0.11428571 0.12857143 0.14285714 0.15714286 0.17142857 0.18571429 0.2 0.21428571 0.22857143 0.24285714 0.25714286 0.27142857 0.28571429 0.3 0.31428571 0.32857143 0.34285714 0.35714286 0.37142857 0.38571429 0.4 0.41428571 0.42857143 0.44285714 0.45714286 0.47142857 0.48571429 0.5 0.51428571 0.52857143 0.54285714 0.55714286 0.57142857 0.58571429 0.6 0.61428571 0.62857143 0.64285714 0.65714286 0.67142857 0.68571429 0.7 0.71428571 0.72857143 0.74285714 0.75714286 0.77142857 0.78571429 0.8 0.81428571 0.82857143 0.84285714 0.85714286 0.87142857 0.88571429 0.9 0.91428571 0.92857143 0.94285714 0.95714286 0.97142857 0.98571429 1 1 1 1 1 1
  arc A14 (-23.84, -68.5668) -> (-22.8468, -69.56) centre (0, -45.72) ccw
  spline S7 degree 5 poles (-22.8468, -69.56) (-22.8333, -69.556) (-22.8062, -69.5481) (-22.7658, -69.536) (-22.7119, -69.5198) (-22.6448, -69.4993) (-22.5778, -69.4785) (-22.5111, -69.4575) (-22.4444, -69.4361) (-22.378, -69.4145) (-22.3118, -69.3927) (-22.2457, -69.3705) (-22.1798, -69.3481) (-22.1141, -69.3254) (-22.0486, -69.3025) (-21.9832, -69.2792) (-21.9181, -69.2557) (-21.8531, -69.2319) (-21.7884, -69.2079) (-21.7238, -69.1835) (-21.6595, -69.1589) (-21.5953, -69.134) (-21.5314, -69.1088) (-21.4676, -69.0833) (-21.4041, -69.0575) (-21.3408, -69.0314) (-21.2777, -69.0051) (-21.2148, -68.9784) (-21.1522, -68.9515) (-21.0897, -68.9243) (-21.0275, -68.8967) (-20.9655, -68.8689) (-20.9038, -68.8408) (-20.8423, -68.8124) (-20.781, -68.7836) (-20.72, -68.7546) (-20.6592, -68.7252) (-20.5987, -68.6956) (-20.5384, -68.6656) (-20.4784, -68.6353) (-20.4187, -68.6047) (-20.3592, -68.5738) (-20.3, -68.5425) (-20.2411, -68.5109) (-20.1825, -68.4789) (-20.1241, -68.4467) (-20.066, -68.4141) (-20.0083, -68.3811) (-19.9508, -68.3479) (-19.8936, -68.3142) (-19.8368, -68.2802) (-19.7803, -68.2458) (-19.7242, -68.2111) (-19.6685, -68.1759) (-19.6131, -68.1403) (-19.558, -68.1043) (-19.5033, -68.068) (-19.4489, -68.0314) (-19.3948, -67.9944) (-19.3412, -67.9569) (-19.288, -67.919) (-19.2355, -67.8804) (-19.1835, -67.8413) (-19.1321, -67.8015) (-19.0813, -67.7612) (-19.0309, -67.7205) (-18.9808, -67.6795) (-18.931, -67.6382) (-18.8816, -67.5965) (-18.8331, -67.554) (-18.7858, -67.5103) (-18.7495, -67.4739) (-18.7233, -67.4457) (-18.7062, -67.4264) (-18.6978, -67.4167) knots -1 -1 -1 -1 -1 -1 -0.98571429 -0.97142857 -0.95714286 -0.94285714 -0.92857143 -0.91428571 -0.9 -0.88571429 -0.87142857 -0.85714286 -0.84285714 -0.82857143 -0.81428571 -0.8 -0.78571429 -0.77142857 -0.75714286 -0.74285714 -0.72857143 -0.71428571 -0.7 -0.68571429 -0.67142857 -0.65714286 -0.64285714 -0.62857143 -0.61428571 -0.6 -0.58571429 -0.57142857 -0.55714286 -0.54285714 -0.52857143 -0.51428571 -0.5 -0.48571429 -0.47142857 -0.45714286 -0.44285714 -0.42857143 -0.41428571 -0.4 -0.38571429 -0.37142857 -0.35714286 -0.34285714 -0.32857143 -0.31428571 -0.3 -0.28571429 -0.27142857 -0.25714286 -0.24285714 -0.22857143 -0.21428571 -0.2 -0.18571429 -0.17142857 -0.15714286 -0.14285714 -0.12857143 -0.11428571 -0.1 -0.08571429 -0.07142857 -0.05714286 -0.04285714 -0.02857143 -0.01428571 0 0 0 0 0 0
  line L7 (-18.6978, -67.4167) -> (-18.685, -67.4019)
  arc A15 (-16.9379, -67.2337) -> (-18.685, -67.4019) centre (-17.7235, -68.2315) ccw
  arc A16 (-16.9379, -67.2337) -> (-16.3968, -67.6489) centre (0, -45.72) ccw
  arc A17 (-16.1071, -69.3801) -> (-16.3968, -67.6489) centre (-17.1573, -68.666) ccw
  line L8 (-16.1071, -69.3801) -> (-16.1181, -69.3962)
  spline S8 degree 5 poles (-16.1181, -69.3962) (-16.1253, -69.4068) (-16.1395, -69.4283) (-16.16, -69.461) (-16.1857, -69.5055) (-16.2157, -69.5624) (-16.2441, -69.6203) (-16.2717, -69.6787) (-16.2986, -69.7375) (-16.3253, -69.7966) (-16.3515, -69.8558) (-16.3773, -69.9153) (-16.4024, -69.9752) (-16.4268, -70.0356) (-16.4504, -70.0963) (-16.4733, -70.1575) (-16.4956, -70.219) (-16.5174, -70.2808) (-16.5387, -70.3428) (-16.5596, -70.4051) (-16.5801, -70.4676) (-16.6001, -70.5303) (-16.6197, -70.5932) (-16.6388, -70.6564) (-16.6574, -70.7199) (-16.6755, -70.7836) (-16.6932, -70.8475) (-16.7105, -70.9116) (-16.7273, -70.976) (-16.7438, -71.0405) (-16.7599, -71.1052) (-16.7755, -71.1701) (-16.7908, -71.2352) (-16.8057, -71.3005) (-16.8202, -71.3659) (-16.8343, -71.4315) (-16.848, -71.4974) (-16.8614, -71.5633) (-16.8743, -71.6295) (-16.887, -71.6958) (-16.8992, -71.7622) (-16.9111, -71.8288) (-16.9227, -71.8956) (-16.9339, -71.9625) (-16.9447, -72.0296) (-16.9552, -72.0968) (-16.9653, -72.1642) (-16.9751, -72.2317) (-16.9846, -72.2993) (-16.9937, -72.3671) (-17.0025, -72.435) (-17.011, -72.503) (-17.0191, -72.5712) (-17.0269, -72.6395) (-17.0343, -72.7079) (-17.0415, -72.7764) (-17.0483, -72.8451) (-17.0548, -72.9138) (-17.0609, -72.9827) (-17.0668, -73.0517) (-17.0723, -73.1209) (-17.0776, -73.1901) (-17.0825, -73.2594) (-17.0871, -73.3289) (-17.0913, -73.3984) (-17.0953, -73.4681) (-17.099, -73.5379) (-17.1023, -73.6077) (-17.1054, -73.6777) (-17.1081, -73.7477) (-17.1106, -73.8179) (-17.1123, -73.8741) (-17.1134, -73.9163) (-17.1142, -73.9444) (-17.1145, -73.9585) knots 0 0 0 0 0 0 0.01428571 0.02857143 0.04285714 0.05714286 0.07142857 0.08571429 0.1 0.11428571 0.12857143 0.14285714 0.15714286 0.17142857 0.18571429 0.2 0.21428571 0.22857143 0.24285714 0.25714286 0.27142857 0.28571429 0.3 0.31428571 0.32857143 0.34285714 0.35714286 0.37142857 0.38571429 0.4 0.41428571 0.42857143 0.44285714 0.45714286 0.47142857 0.48571429 0.5 0.51428571 0.52857143 0.54285714 0.55714286 0.57142857 0.58571429 0.6 0.61428571 0.62857143 0.64285714 0.65714286 0.67142857 0.68571429 0.7 0.71428571 0.72857143 0.74285714 0.75714286 0.77142857 0.78571429 0.8 0.81428571 0.82857143 0.84285714 0.85714286 0.87142857 0.88571429 0.9 0.91428571 0.92857143 0.94285714 0.95714286 0.97142857 0.98571429 1 1 1 1 1 1
  arc A18 (-17.1145, -73.9585) -> (-15.898, -74.6609) centre (0, -45.72) ccw
  spline S9 degree 5 poles (-15.898, -74.6609) (-15.886, -74.6535) (-15.862, -74.6388) (-15.826, -74.6167) (-15.7782, -74.5872) (-15.7187, -74.55) (-15.6594, -74.5125) (-15.6003, -74.4749) (-15.5415, -74.4371) (-15.4829, -74.399) (-15.4246, -74.3608) (-15.3665, -74.3223) (-15.3086, -74.2836) (-15.251, -74.2446) (-15.1937, -74.2055) (-15.1366, -74.1661) (-15.0797, -74.1266) (-15.0232, -74.0868) (-14.9669, -74.0468) (-14.9108, -74.0065) (-14.855, -73.9661) (-14.7995, -73.9254) (-14.7443, -73.8845) (-14.6893, -73.8434) (-14.6346, -73.8021) (-14.5802, -73.7605) (-14.5261, -73.7187) (-14.4722, -73.6767) (-14.4187, -73.6345) (-14.3654, -73.592) (-14.3124, -73.5493) (-14.2598, -73.5064) (-14.2074, -73.4633) (-14.1554, -73.4199) (-14.1036, -73.3763) (-14.0522, -73.3324) (-14.0011, -73.2883) (-13.9503, -73.244) (-13.8998, -73.1995) (-13.8497, -73.1547) (-13.7999, -73.1097) (-13.7505, -73.0644) (-13.7014, -73.0189) (-13.6527, -72.9731) (-13.6043, -72.9271) (-13.5563, -72.8808) (-13.5087, -72.8343) (-13.4614, -72.7875) (-13.4145, -72.7405) (-13.368, -72.6932) (-13.3219, -72.6457) (-13.2762, -72.5978) (-13.231, -72.5497) (-13.1863, -72.5013) (-13.142, -72.4526) (-13.0981, -72.4036) (-13.0546, -72.3544) (-13.0116, -72.3049) (-12.969, -72.2551) (-12.9268, -72.2051) (-12.8853, -72.1547) (-12.8445, -72.1038) (-12.8044, -72.0526) (-12.7651, -72.0008) (-12.7264, -71.9488) (-12.6883, -71.8964) (-12.6505, -71.8438) (-12.6131, -71.791) (-12.5762, -71.738) (-12.5403, -71.6844) (-12.506, -71.6299) (-12.4803, -71.5854) (-12.4622, -71.5514) (-12.4508, -71.5283) (-12.4452, -71.5167) knots -1 -1 -1 -1 -1 -1 -0.98571429 -0.97142857 -0.95714286 -0.94285714 -0.92857143 -0.91428571 -0.9 -0.88571429 -0.87142857 -0.85714286 -0.84285714 -0.82857143 -0.81428571 -0.8 -0.78571429 -0.77142857 -0.75714286 -0.74285714 -0.72857143 -0.71428571 -0.7 -0.68571429 -0.67142857 -0.65714286 -0.64285714 -0.62857143 -0.61428571 -0.6 -0.58571429 -0.57142857 -0.55714286 -0.54285714 -0.52857143 -0.51428571 -0.5 -0.48571429 -0.47142857 -0.45714286 -0.44285714 -0.42857143 -0.41428571 -0.4 -0.38571429 -0.37142857 -0.35714286 -0.34285714 -0.32857143 -0.31428571 -0.3 -0.28571429 -0.27142857 -0.25714286 -0.24285714 -0.22857143 -0.21428571 -0.2 -0.18571429 -0.17142857 -0.15714286 -0.14285714 -0.12857143 -0.11428571 -0.1 -0.08571429 -0.07142857 -0.05714286 -0.04285714 -0.02857143 -0.01428571 0 0 0 0 0 0
  line L9 (-12.4452, -71.5167) -> (-12.4367, -71.4992)
  arc A19 (-10.7926, -70.8845) -> (-12.4367, -71.4992) centre (-11.2931, -72.0517) ccw
  arc A20 (-10.7926, -70.8845) -> (-10.1625, -71.1455) centre (0, -45.72) ccw
  arc A21 (-9.4346, -72.7427) -> (-10.1625, -71.1455) centre (-10.6338, -72.3248) ccw
  line L10 (-9.4346, -72.7427) -> (-9.441, -72.7611)
  spline S10 degree 5 poles (-9.441, -72.7611) (-9.4452, -72.7733) (-9.4534, -72.7977) (-9.4647, -72.8345) (-9.478, -72.8842) (-9.4923, -72.9469) (-9.5048, -73.0102) (-9.5162, -73.0738) (-9.5271, -73.1376) (-9.5375, -73.2015) (-9.5476, -73.2655) (-9.5571, -73.3297) (-9.5658, -73.394) (-9.5738, -73.4586) (-9.5808, -73.5234) (-9.5871, -73.5884) (-9.5927, -73.6536) (-9.5978, -73.7189) (-9.6023, -73.7844) (-9.6064, -73.8499) (-9.61, -73.9156) (-9.6131, -73.9813) (-9.6157, -74.0472) (-9.6178, -74.1132) (-9.6193, -74.1793) (-9.6204, -74.2455) (-9.6209, -74.3118) (-9.621, -74.3782) (-9.6206, -74.4447) (-9.6198, -74.5113) (-9.6186, -74.578) (-9.6169, -74.6447) (-9.6149, -74.7116) (-9.6123, -74.7785) (-9.6094, -74.8454) (-9.606, -74.9125) (-9.6023, -74.9796) (-9.5981, -75.0468) (-9.5935, -75.114) (-9.5885, -75.1813) (-9.5832, -75.2487) (-9.5774, -75.3161) (-9.5713, -75.3836) (-9.5648, -75.4511) (-9.5579, -75.5187) (-9.5506, -75.5864) (-9.543, -75.6541) (-9.535, -75.7218) (-9.5266, -75.7896) (-9.5179, -75.8574) (-9.5088, -75.9253) (-9.4994, -75.9932) (-9.4896, -76.0611) (-9.4794, -76.1291) (-9.4689, -76.1971) (-9.4581, -76.2651) (-9.4469, -76.3332) (-9.4354, -76.4013) (-9.4235, -76.4695) (-9.4113, -76.5376) (-9.3987, -76.6058) (-9.3859, -76.6741) (-9.3727, -76.7423) (-9.3591, -76.8106) (-9.3453, -76.8789) (-9.3311, -76.9472) (-9.3166, -77.0155) (-9.3017, -77.0839) (-9.2866, -77.1522) (-9.2711, -77.2206) (-9.2553, -77.289) (-9.2424, -77.3438) (-9.2326, -77.3848) (-9.226, -77.4122) (-9.2227, -77.4259) knots 0 0 0 0 0 0 0.01428571 0.02857143 0.04285714 0.05714286 0.07142857 0.08571429 0.1 0.11428571 0.12857143 0.14285714 0.15714286 0.17142857 0.18571429 0.2 0.21428571 0.22857143 0.24285714 0.25714286 0.27142857 0.28571429 0.3 0.31428571 0.32857143 0.34285714 0.35714286 0.37142857 0.38571429 0.4 0.41428571 0.42857143 0.44285714 0.45714286 0.47142857 0.48571429 0.5 0.51428571 0.52857143 0.54285714 0.55714286 0.57142857 0.58571429 0.6 0.61428571 0.62857143 0.64285714 0.65714286 0.67142857 0.68571429 0.7 0.71428571 0.72857143 0.74285714 0.75714286 0.77142857 0.78571429 0.8 0.81428571 0.82857143 0.84285714 0.85714286 0.87142857 0.88571429 0.9 0.91428571 0.92857143 0.94285714 0.95714286 0.97142857 0.98571429 1 1 1 1 1 1
  arc A22 (-9.2227, -77.4259) -> (-7.8659, -77.7894) centre (0, -45.72) ccw